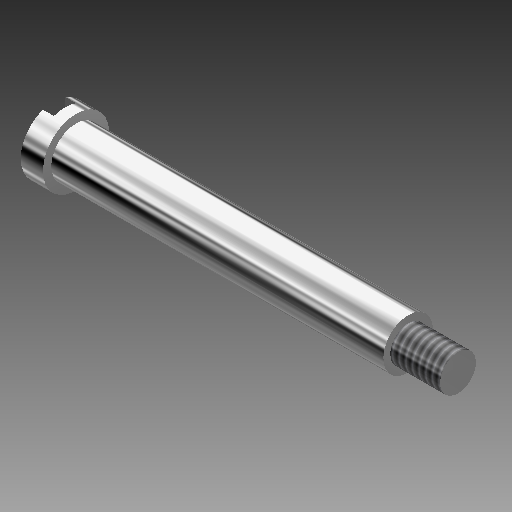
# Autodesk Inventor part: 406-02
Saved by Autodesk Inventor 2019 (Build 230136000, 136)
## iProperties
Company: Autodesk Inc.
Created: 2017-06-27
Part Number: 406-02
Material: Steel, Mild
Document SubType Name: Modeling
Designer: Autodesk Inc.
Mass: 4.39 g
Surface Area: 5.71544 cm^2
Volume: 0.559235 cm^3
Density: 7.85 g/cm^3
Appearance: Chrome - Polished
Author: Inventor
Autodesk Inventor part; units mm, degrees
ref_plane "YZ Plane" through (0, 0, 0) normal (1, 0, 0) x (0, 1, 0)
ref_plane "XZ Plane" through (0, 0, 0) normal (0, 1, 0) x (-1, 0, 0)
ref_plane "XY Plane" through (0, 0, 0) normal (0, 0, 1) x (1, 0, 0)
sketch "Sketch1" plane through (0, 0, 0) normal (0, 0, 1) x (1, 0, 0)
  line L0 (0, 0) -> (2, 0)
  line L1 (2, 0) -> (2, 3)
  line L2 (2, 3) -> (0, 3)
  line L3 (0, 3) -> (0, 0)
  line L4 (2, 0) -> (32, 0)
  line L5 (32, 0) -> (32, 2.25)
  line L6 (32, 2.25) -> (2, 2.25)
  line L7 (2, 2.25) -> (2, 0)
  line L8 (32, 0) -> (36.5, 0)
  line L9 (36.5, 0) -> (36.5, 1.625)
  line L10 (36.5, 1.625) -> (32, 1.625)
  line L11 (32, 1.625) -> (32, 0)
  dimension "d0" = 36.5
  dimension "d1" = 32
  dimension "d2" = 2
  dimension "d3" = 6
  dimension "d4" = 4.5
  dimension "d5" = 3.25
  constraints: 24 end point, 6 parallel, 3 horizontal, 3 perpendicular
  measures "d0" distance between parallel lines of L3 L9
  measures "d1" distance between parallel lines of L5 L3
  measures "d2" distance of L1.end L2.end
  measures "d3" diameter of L2 L0
  measures "d4" diameter of L6 L8
  measures "d5" diameter of L10 L8
revolve "Revolution1" add sketch "Sketch1" angle 360 about axis through (2, 0, 0) along (1, 0, 0)
sketch "Sketch2" plane through (0, 0, 0) normal (0, 1, 0) x (-1, 0, 0)
  line L0 (0, 3) -> (0, -3) projected
  line L1 (-2, 3) -> (-2, -3) projected
  line L2 (0, 1) -> (-1, 1)
  line L3 (-1, 1) -> (-1, -1)
  line L4 (-1, -1) -> (0, -1)
  line L5 (0, -1) -> (0, 1)
  dimension "d10" = 2
  dimension "d11" = 2
  dimension "d12" = 2
  dimension "d15" = 1
  constraints: 8 end point, 2 parallel, 1 horizontal, 1 perpendicular, 1 point on line
  measures "d10" distance of L2.end L3.end
  measures "d11" distance from line of L0.start L2
  measures "d12" distance from line of L0.end L4
  measures "d15" distance of L2.start L2.end
extrude "Extrusion1" cut sketch "Sketch2" along normal mid plane 10
thread "Thread1" size "M3.5x0.6" class "6g" standard "ANSI Metric M Profile" full length
equation "\"d11\" = d12"
body "Solid1"
